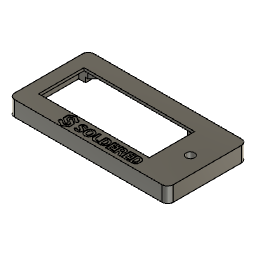
Sensors Case Top (Autodesk Fusion 360 design; units mm, degrees)
Autodesk Fusion 360 part; units mm, degrees
sketch "Sketch1" plane through (0, 0, 0) normal (0, 0, 1) x (1, 0, 0)
  line L0 (65, 35) -> (-65, 35)
  line L1 (-70, 30) -> (-70, -30)
  line L2 (-65, -35) -> (65, -35)
  line L3 (70, -30) -> (70, 30)
  line L4 (70, 35) -> (-70, -35) construction
  line L5 (-70, 35) -> (70, -35) construction
  arc A0 (-65, 35) -> (-70, 30) centre (-65, 30) ccw
  arc A1 (-70, -30) -> (-65, -35) centre (-65, -30) ccw
  arc A2 (65, -35) -> (70, -30) centre (65, -30) ccw
  arc A3 (70, 30) -> (65, 35) centre (65, 30) ccw
  dimension "d1" = 140
  dimension "d2" = 70
  dimension "d3" = 5
  constraint horizontal L0
  constraint perpendicular L0 L1
  constraint parallel L0 L2
  constraint parallel L1 L3
  constraint coincident L4 origin
  constraint coincident L5 origin
  constraint coincident L5.start L0
  constraint coincident L5.start L1
  constraint tangent L0 A0
  constraint tangent L1 A0
  constraint coincident L4.end L1
  constraint coincident L4.end L2
  constraint tangent L1 A1
  constraint tangent L2 A1
  constraint equal A0 A1
  constraint coincident L5.end L3
  constraint coincident L5.end L2
  constraint tangent L3 A2
  constraint tangent L2 A2
  constraint equal A0 A2
  constraint coincident L4.start L3
  constraint coincident L4.start L0
  constraint tangent L3 A3
  constraint tangent L0 A3
  constraint equal A0 A3
  measures "d1" distance of L4.end L5.end
  measures "d2" distance of L5.start L4.end
  measures "d3" radius of A0
extrude "Extrude1" add sketch "Sketch1" along normal blind 14
sketch "Sketch2" plane through (0, 0, 0) normal (0, 0, -1) x (1, 0, 0)
  arc A0 (65, -35) -> (70, -30) centre (65, -30) ccw
  line L0 (70, -30) -> (70, 30)
  arc A1 (70, 30) -> (65, 35) centre (65, 30) ccw
  line L1 (65, 35) -> (-65, 35)
  line L2 (-65, -35) -> (65, -35)
  line L3 (-70, -30) -> (-70, 30)
  line L4 (38.8, 20) -> (-58.8, 20)
  line L5 (-58.8, 20) -> (-58.8, -20)
  line L6 (-58.8, -20) -> (38.8, -20)
  line L7 (38.8, -20) -> (38.8, 20)
  line L8 (38.8, 20) -> (-58.8, -20) construction
  line L9 (-58.8, 20) -> (38.8, -20) construction
  circle A2 centre (-56.6, -27.5) radius 1.6
  circle A3 centre (-56.6, 27.5) radius 2
  circle A4 centre (36.6, 27.5) radius 2
  circle A5 centre (36.6, -27.5) radius 2
  line L10 (39.1, 30) -> (-59.1, 30)
  line L11 (-59.1, 30) -> (-59.1, -30)
  line L12 (-59.1, -30) -> (39.1, -30)
  line L13 (39.1, -30) -> (39.1, 30)
  line L14 (39.1, 30) -> (-59.1, -30) construction
  line L15 (-59.1, 30) -> (39.1, -30) construction
  point P0 (-10, 0)
  point P1 (-10, 0)
  dimension "d70" = 97.6
  dimension "d71" = 40
  dimension "d72" = 3.2
  dimension "d76" = 4
  dimension "d79" = 4
  dimension "d82" = 4
  dimension "d115" = 60
  dimension "d116" = 98.2
  dimension "d117" = 60
  dimension "d118" = 2.5
  dimension "d119" = 2.5
  dimension "d120" = 2.5
  dimension "d121" = 2.5
  dimension "d122" = 2.5
  dimension "d123" = 2.5
  dimension "d124" = 2.5
  dimension "d125" = 2.5
  constraint horizontal L4
  constraint perpendicular L4 L5
  constraint parallel L4 L6
  constraint parallel L5 L7
  constraint coincident L8 P1
  constraint coincident L9 P1
  constraint horizontal L10
  constraint perpendicular L10 L11
  constraint parallel L10 L12
  constraint parallel L11 L13
  constraint coincident L14 P1
  constraint coincident L15 P1
  constraint coincident P1 P0
  measures "d70" distance of L5.end L6.end
  measures "d71" distance of L4.end L5.end
  measures "d72" diameter of A2
  measures "d76" diameter of A3
  measures "d79" diameter of A4
  measures "d82" diameter of A5
  measures "d115" distance of L3 P1
  measures "d116" distance of L11.end L12.end
  measures "d117" distance of L10.end L11.end
  measures "d118" distance of A4.centre L10
  measures "d119" distance of A4.centre L13
  measures "d120" distance of A3.centre L10
  measures "d121" distance of A3.centre L11
  measures "d122" distance of A2.centre L11
  measures "d123" distance of A2.centre L12
  measures "d124" distance of A5.centre L13
  measures "d125" distance of A5.centre L12
extrude "Extrude2" cut sketch "Sketch2" against normal blind 14 contours L4 L5 L6 L7
extrude "Extrude3" cut sketch "Sketch2" against normal blind 8 contours A3 | A4 | A5
sketch "Sketch3" plane through (0, 0, 0) normal (0, 0, -1) x (1, 0, 0)
  arc A0 (65, -35) -> (70, -30) centre (65, -30) ccw
  line L0 (70, -30) -> (70, 30)
  arc A1 (70, 30) -> (65, 35) centre (65, 30) ccw
  line L1 (65, 35) -> (-65, 35)
  arc A2 (-65, 35) -> (-70, 30) centre (-65, 30) ccw
  line L2 (-70, 30) -> (-70, -30)
  arc A3 (-70, -30) -> (-65, -35) centre (-65, -30) ccw
  line L3 (-65, -35) -> (65, -35)
  line L4 (-66, 40) -> (-66, -43.0482) construction
  line L5 (-75, 31) -> (85, 31) construction
  line L6 (66, 43.2494) -> (66, -50) construction
  line L7 (77.8761, -31) -> (-86.4807, -31) construction
  circle A4 centre (-66, -31) radius 2
  circle A5 centre (-66, 31) radius 2
  circle A6 centre (66, 31) radius 2
  circle A7 centre (66, -31) radius 2
  line L8 (38.8, 20) -> (38.8, -20)
  line L9 (38.8, -20) -> (-58.8, -20)
  circle A8 centre (36.6, -27.5) radius 2
  circle A9 centre (36.6, 27.5) radius 2
  circle A10 centre (-56.6, 27.5) radius 2
  line L10 (-58.8, 20) -> (38.8, 20)
  line L11 (-58.8, -20) -> (-58.8, 20)
  dimension "d24" = 4
  dimension "d25" = 4
  dimension "d26" = 4
  dimension "d27" = 4
  dimension "d28" = 4
  dimension "d29" = 4
  dimension "d30" = 4
  dimension "d31" = 4
  constraint perpendicular L1 L4
  constraint perpendicular L4 L5
  constraint perpendicular L3 L6
  constraint perpendicular L6 L7
  constraint coincident L7 A4.centre
  constraint coincident L4 A4.centre
  constraint coincident L4 A5.centre
  constraint coincident L5 A5.centre
  constraint coincident L5 A6.centre
  constraint coincident L6 A6.centre
  constraint coincident L6 A7.centre
  constraint coincident L7 A7.centre
  measures "d24" distance of L2 L4
  measures "d25" distance of L1 L5
  measures "d26" distance of L0 L6
  measures "d27" distance of L3 L7
  measures "d28" diameter of A4
  measures "d29" diameter of A5
  measures "d30" diameter of A6
  measures "d31" diameter of A7
extrude "Extrude4" cut sketch "Sketch3" against normal blind 4 contours A4 | A5 | A6 | A7
sketch "Sketch4" plane through (0, 0, 14) normal (0, 0, 1) x (-1, 0, 0)
  arc A0 (-70, -30) -> (-65, -35) centre (-65, -30) ccw
  line L0 (-65, -35) -> (65, -35)
  arc A1 (65, -35) -> (70, -30) centre (65, -30) ccw
  line L1 (70, -30) -> (70, 30)
  arc A2 (70, 30) -> (65, 35) centre (65, 30) ccw
  line L2 (65, 35) -> (-65, 35)
  arc A3 (-65, 35) -> (-70, 30) centre (-65, 30) ccw
  line L3 (-70, 30) -> (-70, -30)
  circle A4 centre (-55, 0) radius 3.75
  line L4 (-38.8, 20) -> (58.8, 20)
  line L5 (58.8, 20) -> (58.8, -20)
  line L6 (58.8, -20) -> (-38.8, -20)
  line L7 (-38.8, -20) -> (-38.8, 20)
  dimension "d34" = 7.5
  measures "d34" diameter of A4
extrude "Extrude5" cut sketch "Sketch4" against normal blind 10 contours A4
sketch "Sketch5" plane through (0, 0, 0) normal (0, 0, -1) x (1, 0, 0)
  circle A0 centre (66, -31) radius 2
  circle A1 centre (-66, -31) radius 2
  circle A2 centre (66, 31) radius 2
  circle A3 centre (-66, 31) radius 2
  arc A4 (65, -35) -> (70, -30) centre (65, -30) ccw
  line L0 (70, -30) -> (70, 30)
  arc A5 (70, 30) -> (65, 35) centre (65, 30) ccw
  line L1 (65, 35) -> (-65, 35)
  arc A6 (-65, 35) -> (-70, 30) centre (-65, 30) ccw
  line L2 (-70, 30) -> (-70, -30)
  arc A7 (-70, -30) -> (-65, -35) centre (-65, -30) ccw
  line L3 (-65, -35) -> (65, -35)
  line L4 (63, 8) -> (47, 8)
  line L5 (47, 8) -> (47, -8)
  line L6 (47, -8) -> (63, -8)
  line L7 (63, -8) -> (63, 8)
  line L8 (63, 8) -> (47, -8) construction
  line L9 (47, 8) -> (63, -8) construction
  line L10 (38.8, 20) -> (38.8, -20)
  line L11 (38.8, -20) -> (-58.8, -20)
  circle A8 centre (36.6, -27.5) radius 2
  circle A9 centre (36.6, 27.5) radius 2
  circle A10 centre (-56.6, 27.5) radius 2
  line L12 (-58.8, 20) -> (38.8, 20)
  line L13 (-58.8, -20) -> (-58.8, 20)
  point P0 (55, 0)
  dimension "d37" = 16
  dimension "d38" = 16
  constraint horizontal L4
  constraint perpendicular L4 L5
  constraint parallel L4 L6
  constraint parallel L5 L7
  constraint coincident L8 P0
  constraint coincident L9 P0
  measures "d37" distance of L5.end L6.end
  measures "d38" distance of L4.end L5.end
extrude "Extrude6" cut sketch "Sketch5" against normal blind 7 contours L4 L5 L6 L7
chamfer "Chamfer1" distance 2 angle 45 4 edges at (55, -8, 0) (63, 0, 0) (47, 0, 0) (55, 8, 0)
extrude "Extrude7" cut 1 faces at (54.6934, -17.9132, 14) along direction (0, 0, -1) blind 0.6
sketch "Sketch6" plane through (0, 0, 13.4) normal (0, 0, 1) x (-1, 0, 0)
  circle A0 centre (-55, 0) radius 3.75
  arc A1 (-70, -30) -> (-65, -35) centre (-65, -30) ccw
  line L0 (-65, -35) -> (65, -35)
  arc A2 (65, -35) -> (70, -30) centre (65, -30) ccw
  line L1 (70, -30) -> (70, 30)
  arc A3 (70, 30) -> (65, 35) centre (65, 30) ccw
  line L2 (65, 35) -> (-65, 35)
  arc A4 (-65, 35) -> (-70, 30) centre (-65, 30) ccw
  line L3 (-70, 30) -> (-70, -30)
  spline S0 degree 3 poles (14.0223, 31.6995) (14.566, 31.6995) (15.1035, 31.6031) (15.6345, 31.4109) knots 0 0 0 0 1 1 1 1
  spline S1 degree 3 poles (15.6345, 31.4109) (16.1658, 31.2184) (16.649, 30.9174) (17.0838, 30.5076) knots 0 0 0 0 1 1 1 1
  line L4 (17.0838, 30.5076) -> (16.0297, 29.2151)
  spline S2 degree 3 poles (16.0297, 29.2151) (15.737, 29.4578) (15.4068, 29.6438) (15.0385, 29.7734) knots 0 0 0 0 1 1 1 1
  spline S3 degree 3 poles (15.0385, 29.7734) (14.6706, 29.9032) (14.3152, 29.9679) (13.9721, 29.9679) knots 0 0 0 0 1 1 1 1
  spline S4 degree 3 poles (13.9721, 29.9679) (13.6207, 29.9679) (13.3594, 29.9095) (13.1877, 29.7924) knots 0 0 0 0 1 1 1 1
  spline S5 degree 3 poles (13.1877, 29.7924) (13.0165, 29.6752) (12.9306, 29.508) (12.9306, 29.2905) knots 0 0 0 0 1 1 1 1
  spline S6 degree 3 poles (12.9306, 29.2905) (12.9306, 29.1315) (12.9787, 29.0062) (13.0749, 28.9139) knots 0 0 0 0 1 1 1 1
  spline S7 degree 3 poles (13.0749, 28.9139) (13.1712, 28.822) (13.3028, 28.7384) (13.4703, 28.6631) knots 0 0 0 0 1 1 1 1
  spline S8 degree 3 poles (13.4703, 28.6631) (13.6376, 28.5877) (13.8382, 28.5043) (14.0723, 28.412) knots 0 0 0 0 1 1 1 1
  line L5 (14.0723, 28.412) -> (15.1139, 27.973)
  spline S9 degree 3 poles (15.1139, 27.973) (15.4068, 27.8557) (15.6784, 27.6968) (15.9295, 27.4962) knots 0 0 0 0 1 1 1 1
  spline S10 degree 3 poles (15.9295, 27.4962) (16.1803, 27.2954) (16.3833, 27.0465) (16.538, 26.7496) knots 0 0 0 0 1 1 1 1
  spline S11 degree 3 poles (16.538, 26.7496) (16.6928, 26.4528) (16.77, 26.1076) (16.77, 25.7143) knots 0 0 0 0 1 1 1 1
  spline S12 degree 3 poles (16.77, 25.7143) (16.77, 25.2544) (16.6426, 24.8383) (16.3873, 24.4661) knots 0 0 0 0 1 1 1 1
  spline S13 degree 3 poles (16.3873, 24.4661) (16.1324, 24.0937) (15.7811, 23.7947) (15.3335, 23.5687) knots 0 0 0 0 1 1 1 1
  spline S14 degree 3 poles (15.3335, 23.5687) (14.8861, 23.3431) (14.3695, 23.2299) (13.7839, 23.2299) knots 0 0 0 0 1 1 1 1
  spline S15 degree 3 poles (13.7839, 23.2299) (13.2904, 23.2299) (12.8113, 23.3179) (12.3473, 23.4935) knots 0 0 0 0 1 1 1 1
  spline S16 degree 3 poles (12.3473, 23.4935) (11.8829, 23.6691) (11.475, 23.9243) (11.1238, 24.2588) knots 0 0 0 0 1 1 1 1
  line L6 (11.1238, 24.2588) -> (12.1651, 25.5639)
  spline S17 degree 3 poles (12.1651, 25.5639) (12.4413, 25.363) (12.7152, 25.2124) (12.987, 25.1122) knots 0 0 0 0 1 1 1 1
  spline S18 degree 3 poles (12.987, 25.1122) (13.259, 25.0118) (13.5247, 24.9616) (13.7839, 24.9616) knots 0 0 0 0 1 1 1 1
  spline S19 degree 3 poles (13.7839, 24.9616) (14.0766, 24.9616) (14.3089, 25.0161) (14.4801, 25.1246) knots 0 0 0 0 1 1 1 1
  spline S20 degree 3 poles (14.4801, 25.1246) (14.6518, 25.2335) (14.7376, 25.3925) (14.7376, 25.6014) knots 0 0 0 0 1 1 1 1
  spline S21 degree 3 poles (14.7376, 25.6014) (14.7376, 25.7437) (14.6873, 25.865) (14.5869, 25.9654) knots 0 0 0 0 1 1 1 1
  spline S22 degree 3 poles (14.5869, 25.9654) (14.4865, 26.0658) (14.3422, 26.1535) (14.154, 26.2289) knots 0 0 0 0 1 1 1 1
  spline S23 degree 3 poles (14.154, 26.2289) (13.9657, 26.3042) (13.7505, 26.3919) (13.5078, 26.4924) knots 0 0 0 0 1 1 1 1
  line L7 (13.5078, 26.4924) -> (12.4916, 26.8938)
  spline S24 degree 3 poles (12.4916, 26.8938) (12.157, 27.0277) (11.8704, 27.1972) (11.632, 27.402) knots 0 0 0 0 1 1 1 1
  spline S25 degree 3 poles (11.632, 27.402) (11.3936, 27.607) (11.2098, 27.8497) (11.0799, 28.1297) knots 0 0 0 0 1 1 1 1
  spline S26 degree 3 poles (11.0799, 28.1297) (10.9503, 28.4102) (10.8854, 28.7427) (10.8854, 29.1271) knots 0 0 0 0 1 1 1 1
  spline S27 degree 3 poles (10.8854, 29.1271) (10.8854, 29.5875) (11.0066, 30.0118) (11.2493, 30.4008) knots 0 0 0 0 1 1 1 1
  spline S28 degree 3 poles (11.2493, 30.4008) (11.492, 30.7898) (11.8474, 31.1036) (12.3157, 31.342) knots 0 0 0 0 1 1 1 1
  spline S29 degree 3 poles (12.3157, 31.342) (12.7845, 31.5804) (13.3531, 31.6995) (14.0223, 31.6995) knots 0 0 0 0 1 1 1 1
  spline S30 degree 3 poles (6.5316, 29.9679) (6.1801, 29.9679) (5.8771, 29.8657) (5.6219, 29.6605) knots 0 0 0 0 1 1 1 1
  spline S31 degree 3 poles (5.6219, 29.6605) (5.3668, 29.4556) (5.1723, 29.163) (5.0384, 28.7822) knots 0 0 0 0 1 1 1 1
  spline S32 degree 3 poles (5.0384, 28.7822) (4.9046, 28.4016) (4.8377, 27.9521) (4.8377, 27.4333) knots 0 0 0 0 1 1 1 1
  spline S33 degree 3 poles (4.8377, 27.4333) (4.8377, 26.9063) (4.9046, 26.4609) (5.0384, 26.097) knots 0 0 0 0 1 1 1 1
  spline S34 degree 3 poles (5.0384, 26.097) (5.1723, 25.7333) (5.3668, 25.4531) (5.6219, 25.2563) knots 0 0 0 0 1 1 1 1
  spline S35 degree 3 poles (5.6219, 25.2563) (5.8771, 25.06) (6.1801, 24.9616) (6.5316, 24.9616) knots 0 0 0 0 1 1 1 1
  spline S36 degree 3 poles (6.5316, 24.9616) (6.8829, 24.9616) (7.1862, 25.06) (7.4413, 25.2563) knots 0 0 0 0 1 1 1 1
  spline S37 degree 3 poles (7.4413, 25.2563) (7.6964, 25.4531) (7.8909, 25.7333) (8.0247, 26.097) knots 0 0 0 0 1 1 1 1
  spline S38 degree 3 poles (8.0247, 26.097) (8.1586, 26.4609) (8.2255, 26.9063) (8.2255, 27.4333) knots 0 0 0 0 1 1 1 1
  spline S39 degree 3 poles (8.2255, 27.4333) (8.2255, 27.9521) (8.1586, 28.4016) (8.0247, 28.7822) knots 0 0 0 0 1 1 1 1
  spline S40 degree 3 poles (8.0247, 28.7822) (7.8909, 29.163) (7.6964, 29.4556) (7.4413, 29.6605) knots 0 0 0 0 1 1 1 1
  spline S41 degree 3 poles (7.4413, 29.6605) (7.1862, 29.8657) (6.8829, 29.9679) (6.5316, 29.9679) knots 0 0 0 0 1 1 1 1
  spline S42 degree 3 poles (6.5316, 31.6996) (7.2762, 31.6996) (7.9305, 31.5301) (8.4953, 31.1913) knots 0 0 0 0 1 1 1 1
  spline S43 degree 3 poles (8.4953, 31.1913) (9.0598, 30.8525) (9.4989, 30.3632) (9.8126, 29.7232) knots 0 0 0 0 1 1 1 1
  spline S44 degree 3 poles (9.8126, 29.7232) (10.1263, 29.0833) (10.2833, 28.3201) (10.2833, 27.4333) knots 0 0 0 0 1 1 1 1
  spline S45 degree 3 poles (10.2833, 27.4333) (10.2833, 26.5383) (10.1263, 25.7792) (9.8126, 25.1561) knots 0 0 0 0 1 1 1 1
  spline S46 degree 3 poles (9.8126, 25.1561) (9.4989, 24.533) (9.0598, 24.0561) (8.4953, 23.7257) knots 0 0 0 0 1 1 1 1
  spline S47 degree 3 poles (8.4953, 23.7257) (7.9305, 23.3953) (7.2762, 23.2299) (6.5316, 23.2299) knots 0 0 0 0 1 1 1 1
  spline S48 degree 3 poles (6.5316, 23.2299) (5.7872, 23.2299) (5.1325, 23.3953) (4.5678, 23.7257) knots 0 0 0 0 1 1 1 1
  spline S49 degree 3 poles (4.5678, 23.7257) (4.0034, 24.0561) (3.5641, 24.533) (3.2503, 25.1561) knots 0 0 0 0 1 1 1 1
  spline S50 degree 3 poles (3.2503, 25.1561) (2.9367, 25.7792) (2.7799, 26.5383) (2.7799, 27.4333) knots 0 0 0 0 1 1 1 1
  spline S51 degree 3 poles (2.7799, 27.4333) (2.7799, 28.3201) (2.9367, 29.0833) (3.2503, 29.7232) knots 0 0 0 0 1 1 1 1
  spline S52 degree 3 poles (3.2503, 29.7232) (3.5641, 30.3632) (4.0034, 30.8525) (4.5678, 31.1913) knots 0 0 0 0 1 1 1 1
  spline S53 degree 3 poles (4.5678, 31.1913) (5.1325, 31.5301) (5.7872, 31.6996) (6.5316, 31.6996) knots 0 0 0 0 1 1 1 1
  line L8 (-6.2916, 29.9428) -> (-6.53, 29.9428)
  spline S54 degree 3 poles (-6.53, 29.9428) (-6.9565, 29.9428) (-7.3373, 29.8675) (-7.6717, 29.7171) knots 0 0 0 0 1 1 1 1
  spline S55 degree 3 poles (-7.6717, 29.7171) (-8.0063, 29.5665) (-8.2698, 29.3093) (-8.4623, 28.9452) knots 0 0 0 0 1 1 1 1
  spline S56 degree 3 poles (-8.4623, 28.9452) (-8.6546, 28.5814) (-8.7508, 28.0777) (-8.7508, 27.4332) knots 0 0 0 0 1 1 1 1
  spline S57 degree 3 poles (-8.7508, 27.4332) (-8.7508, 26.7894) (-8.6546, 26.2916) (-8.4623, 25.9403) knots 0 0 0 0 1 1 1 1
  spline S58 degree 3 poles (-8.4623, 25.9403) (-8.2698, 25.589) (-8.0063, 25.3422) (-7.6717, 25.2) knots 0 0 0 0 1 1 1 1
  spline S59 degree 3 poles (-7.6717, 25.2) (-7.3373, 25.0577) (-6.9565, 24.9867) (-6.53, 24.9867) knots 0 0 0 0 1 1 1 1
  line L9 (-6.53, 24.9867) -> (-6.2916, 24.9867)
  line L10 (-6.2916, 24.9867) -> (-6.2916, 29.9428)
  line L11 (-4.284, 31.5489) -> (-4.284, 23.3806)
  line L12 (-4.284, 23.3806) -> (-6.6555, 23.3806)
  spline S60 degree 3 poles (-6.6555, 23.3806) (-7.4836, 23.3806) (-8.2092, 23.5208) (-8.8325, 23.8008) knots 0 0 0 0 1 1 1 1
  spline S61 degree 3 poles (-8.8325, 23.8008) (-9.4555, 24.0812) (-9.9386, 24.5182) (-10.2818, 25.1122) knots 0 0 0 0 1 1 1 1
  spline S62 degree 3 poles (-10.2818, 25.1122) (-10.6246, 25.7062) (-10.796, 26.4797) (-10.796, 27.4332) knots 0 0 0 0 1 1 1 1
  spline S63 degree 3 poles (-10.796, 27.4332) (-10.796, 28.3787) (-10.6246, 29.1546) (-10.2818, 29.761) knots 0 0 0 0 1 1 1 1
  spline S64 degree 3 poles (-10.2818, 29.761) (-9.9386, 30.3675) (-9.4641, 30.817) (-8.8576, 31.1097) knots 0 0 0 0 1 1 1 1
  spline S65 degree 3 poles (-8.8576, 31.1097) (-8.251, 31.4026) (-7.5547, 31.5489) (-6.7684, 31.5489) knots 0 0 0 0 1 1 1 1
  line L13 (-6.7684, 31.5489) -> (-4.284, 31.5489)
  line L14 (-11.7133, 31.5489) -> (-11.7133, 23.3806)
  line L15 (-11.7133, 23.3806) -> (-16.9204, 23.3806)
  line L16 (-16.9204, 23.3806) -> (-16.9204, 25.0619)
  line L17 (-16.9204, 25.0619) -> (-13.7209, 25.0619)
  line L18 (-13.7209, 25.0619) -> (-13.7209, 26.5174)
  line L19 (-13.7209, 26.5174) -> (-16.4437, 26.5174)
  line L20 (-16.4437, 26.5174) -> (-16.4437, 28.1987)
  line L21 (-16.4437, 28.1987) -> (-13.7209, 28.1987)
  line L22 (-13.7209, 28.1987) -> (-13.7209, 29.8675)
  line L23 (-13.7209, 29.8675) -> (-17.0459, 29.8675)
  line L24 (-17.0459, 29.8675) -> (-17.0459, 31.5489)
  line L25 (-17.0459, 31.5489) -> (-11.7133, 31.5489)
  line L26 (-20.145, 24.974) -> (-21.0109, 24.974)
  spline S66 degree 3 poles (-21.0109, 24.974) (-21.4625, 24.974) (-21.8074, 25.0452) (-22.0458, 25.1873) knots 0 0 0 0 1 1 1 1
  spline S67 degree 3 poles (-22.0458, 25.1873) (-22.2843, 25.3297) (-22.4035, 25.5933) (-22.4035, 25.9778) knots 0 0 0 0 1 1 1 1
  spline S68 degree 3 poles (-22.4035, 25.9778) (-22.4035, 26.3544) (-22.2843, 26.6388) (-22.0458, 26.8312) knots 0 0 0 0 1 1 1 1
  spline S69 degree 3 poles (-22.0458, 26.8312) (-21.8074, 27.0237) (-21.4625, 27.1196) (-21.0109, 27.1196) knots 0 0 0 0 1 1 1 1
  line L27 (-21.0109, 27.1196) -> (-20.145, 27.1196)
  line L28 (-20.145, 27.1196) -> (-20.145, 24.974)
  line L29 (-24.7876, 31.5489) -> (-22.974, 28.3209)
  spline S70 degree 3 poles (-22.974, 28.3209) (-23.3572, 28.1311) (-23.678, 27.8717) (-23.9282, 27.5337) knots 0 0 0 0 1 1 1 1
  spline S71 degree 3 poles (-23.9282, 27.5337) (-24.225, 27.1323) (-24.3736, 26.6136) (-24.3736, 25.9778) knots 0 0 0 0 1 1 1 1
  spline S72 degree 3 poles (-24.3736, 25.9778) (-24.3736, 25.3088) (-24.225, 24.7858) (-23.9282, 24.4094) knots 0 0 0 0 1 1 1 1
  spline S73 degree 3 poles (-23.9282, 24.4094) (-23.631, 24.0331) (-23.2399, 23.7676) (-22.7549, 23.6127) knots 0 0 0 0 1 1 1 1
  spline S74 degree 3 poles (-22.7549, 23.6127) (-22.2696, 23.4579) (-21.7385, 23.3806) (-21.1615, 23.3806) knots 0 0 0 0 1 1 1 1
  line L30 (-21.1615, 23.3806) -> (-18.1375, 23.3806)
  line L31 (-18.1375, 23.3806) -> (-18.1375, 31.5489)
  line L32 (-18.1375, 31.5489) -> (-20.145, 31.5489)
  line L33 (-20.145, 31.5489) -> (-20.145, 28.7133)
  line L34 (-20.145, 28.7133) -> (-21.0729, 28.7133)
  line L35 (-21.0729, 28.7133) -> (-22.5541, 31.5489)
  line L36 (-22.5541, 31.5489) -> (-24.7876, 31.5489)
  line L37 (-25.5653, 31.5489) -> (-25.5653, 23.3806)
  line L38 (-25.5653, 23.3806) -> (-30.7725, 23.3806)
  line L39 (-30.7725, 23.3806) -> (-30.7725, 25.0619)
  line L40 (-30.7725, 25.0619) -> (-27.5728, 25.0619)
  line L41 (-27.5728, 25.0619) -> (-27.5728, 26.5174)
  line L42 (-27.5728, 26.5174) -> (-30.2957, 26.5174)
  line L43 (-30.2957, 26.5174) -> (-30.2957, 28.1987)
  line L44 (-30.2957, 28.1987) -> (-27.5728, 28.1987)
  line L45 (-27.5728, 28.1987) -> (-27.5728, 29.8675)
  line L46 (-27.5728, 29.8675) -> (-30.8979, 29.8675)
  line L47 (-30.8979, 29.8675) -> (-30.8979, 31.5489)
  line L48 (-30.8979, 31.5489) -> (-25.5653, 31.5489)
  line L49 (-33.8716, 29.9428) -> (-34.11, 29.9428)
  spline S75 degree 3 poles (-34.11, 29.9428) (-34.5366, 29.9428) (-34.9173, 29.8675) (-35.2518, 29.7171) knots 0 0 0 0 1 1 1 1
  spline S76 degree 3 poles (-35.2518, 29.7171) (-35.5863, 29.5665) (-35.8499, 29.3093) (-36.0423, 28.9452) knots 0 0 0 0 1 1 1 1
  spline S77 degree 3 poles (-36.0423, 28.9452) (-36.2346, 28.5814) (-36.3309, 28.0777) (-36.3309, 27.4332) knots 0 0 0 0 1 1 1 1
  spline S78 degree 3 poles (-36.3309, 27.4332) (-36.3309, 26.7894) (-36.2346, 26.2916) (-36.0423, 25.9403) knots 0 0 0 0 1 1 1 1
  spline S79 degree 3 poles (-36.0423, 25.9403) (-35.8499, 25.589) (-35.5863, 25.3422) (-35.2518, 25.2) knots 0 0 0 0 1 1 1 1
  spline S80 degree 3 poles (-35.2518, 25.2) (-34.9173, 25.0577) (-34.5366, 24.9867) (-34.11, 24.9867) knots 0 0 0 0 1 1 1 1
  line L50 (-34.11, 24.9867) -> (-33.8716, 24.9867)
  line L51 (-33.8716, 24.9867) -> (-33.8716, 29.9428)
  line L52 (-31.8641, 31.5489) -> (-31.8641, 23.3806)
  line L53 (-31.8641, 23.3806) -> (-34.2355, 23.3806)
  spline S81 degree 3 poles (-34.2355, 23.3806) (-35.0636, 23.3806) (-35.7892, 23.5208) (-36.4126, 23.8008) knots 0 0 0 0 1 1 1 1
  spline S82 degree 3 poles (-36.4126, 23.8008) (-37.0355, 24.0812) (-37.5186, 24.5182) (-37.8618, 25.1122) knots 0 0 0 0 1 1 1 1
  spline S83 degree 3 poles (-37.8618, 25.1122) (-38.2046, 25.7062) (-38.376, 26.4797) (-38.376, 27.4332) knots 0 0 0 0 1 1 1 1
  spline S84 degree 3 poles (-38.376, 27.4332) (-38.376, 28.3787) (-38.2046, 29.1546) (-37.8618, 29.761) knots 0 0 0 0 1 1 1 1
  spline S85 degree 3 poles (-37.8618, 29.761) (-37.5186, 30.3675) (-37.0441, 30.817) (-36.4376, 31.1097) knots 0 0 0 0 1 1 1 1
  spline S86 degree 3 poles (-36.4376, 31.1097) (-35.831, 31.4026) (-35.1347, 31.5489) (-34.3485, 31.5489) knots 0 0 0 0 1 1 1 1
  line L54 (-34.3485, 31.5489) -> (-31.8641, 31.5489)
  line L55 (-1.2206, 29.5917) -> (-0.0935, 28.4645)
  line L56 (-0.0935, 28.4645) -> (-0.0935, 23.3806)
  line L57 (-0.0935, 23.3806) -> (1.9141, 23.3806)
  line L58 (1.9141, 23.3806) -> (1.9141, 29.4411)
  line L59 (1.9141, 29.4411) -> (-0.1704, 31.5255)
  line L60 (-0.1704, 31.5255) -> (-3.3165, 31.5255)
  line L61 (-3.3165, 31.5255) -> (-3.3165, 29.5917)
  line L62 (-3.3165, 29.5917) -> (-1.2206, 29.5917)
  line L63 (21.169, 22.4657) -> (21.1725, 22.4657)
  spline S87 degree 3 poles (21.1725, 22.4657) (21.4299, 22.4663) (21.6835, 22.4038) (21.9065, 22.2751) knots 0 0 0 0 1 1 1 1
  line L64 (21.9065, 22.2751) -> (25.0192, 20.478)
  line L65 (25.0192, 20.478) -> (29.6844, 23.1693)
  line L66 (29.6844, 23.1693) -> (29.6844, 27.7005)
  line L67 (29.6844, 27.7005) -> (24.7789, 30.5327)
  line L68 (24.7789, 30.5327) -> (24.665, 30.4733)
  spline S88 degree 3 poles (24.665, 30.4733) (24.2399, 30.2534) (23.9257, 29.7858) (23.919, 29.3072) knots 0 0 0 0 1 1 1 1
  spline S89 degree 3 poles (23.919, 29.3072) (23.9121, 28.8287) (24.2143, 28.292) (24.6326, 28.0603) knots 0 0 0 0 1 1 1 1
  line L69 (24.6326, 28.0603) -> (27.5947, 26.4695)
  line L70 (27.5947, 26.4695) -> (27.5947, 24.3462)
  line L71 (27.5947, 24.3462) -> (25.0293, 22.8515)
  line L72 (25.0293, 22.8515) -> (22.8789, 24.1087)
  spline S90 degree 3 poles (22.8789, 24.1087) (22.6755, 24.2276) (22.5102, 24.3999) (22.3905, 24.6028) knots 0 0 0 0 1 1 1 1
  spline S91 degree 3 poles (22.3905, 24.6028) (22.1439, 25.0206) (21.6892, 25.301) (21.169, 25.301) knots 0 0 0 0 1 1 1 1
  spline S92 degree 3 poles (21.169, 25.301) (20.6954, 25.301) (20.2764, 25.0686) (20.0189, 24.7118) knots 0 0 0 0 1 1 1 1
  spline S93 degree 3 poles (20.0189, 24.7118) (19.9943, 24.6789) (19.971, 24.6443) (19.95, 24.6077) knots 0 0 0 0 1 1 1 1
  spline S94 degree 3 poles (19.95, 24.6077) (19.9472, 24.603) (19.9448, 24.5983) (19.9423, 24.5935) knots 0 0 0 0 1 1 1 1
  spline S95 degree 3 poles (19.9423, 24.5935) (19.8211, 24.3846) (19.7514, 24.1422) (19.7514, 23.8833) knots 0 0 0 0 1 1 1 1
  spline S96 degree 3 poles (19.7514, 23.8833) (19.7514, 23.1005) (20.386, 22.4657) (21.169, 22.4657) knots 0 0 0 0 1 1 1 1
  spline S97 degree 3 poles (25.2044, 24.2526) (25.6294, 24.4726) (25.9437, 24.9401) (25.9505, 25.4187) knots 0 0 0 0 1 1 1 1
  spline S98 degree 3 poles (25.9505, 25.4187) (25.9573, 25.8972) (25.6551, 26.434) (25.2368, 26.6656) knots 0 0 0 0 1 1 1 1
  line L73 (25.2368, 26.6656) -> (22.2747, 28.2565)
  line L74 (22.2747, 28.2565) -> (22.2747, 30.3797)
  line L75 (22.2747, 30.3797) -> (24.8401, 31.8744)
  line L76 (24.8401, 31.8744) -> (26.9905, 30.6172)
  spline S99 degree 3 poles (26.9905, 30.6172) (27.1939, 30.4984) (27.3593, 30.3262) (27.4789, 30.1232) knots 0 0 0 0 1 1 1 1
  spline S100 degree 3 poles (27.4789, 30.1232) (27.7255, 29.7053) (28.1801, 29.425) (28.7004, 29.425) knots 0 0 0 0 1 1 1 1
  spline S101 degree 3 poles (28.7004, 29.425) (29.174, 29.425) (29.593, 29.6574) (29.8504, 30.0141) knots 0 0 0 0 1 1 1 1
  spline S102 degree 3 poles (29.8504, 30.0141) (29.8751, 30.0471) (29.8983, 30.0816) (29.9194, 30.1182) knots 0 0 0 0 1 1 1 1
  spline S103 degree 3 poles (29.9194, 30.1182) (29.9222, 30.123) (29.9245, 30.1277) (29.9271, 30.1323) knots 0 0 0 0 1 1 1 1
  spline S104 degree 3 poles (29.9271, 30.1323) (30.0483, 30.3413) (30.118, 30.5837) (30.118, 30.8426) knots 0 0 0 0 1 1 1 1
  spline S105 degree 3 poles (30.118, 30.8426) (30.118, 31.6256) (29.4833, 32.2602) (28.7004, 32.2602) knots 0 0 0 0 1 1 1 1
  line L77 (28.7004, 32.2602) -> (28.697, 32.2602)
  spline S106 degree 3 poles (28.697, 32.2602) (28.4394, 32.2596) (28.1858, 32.3221) (27.9629, 32.4508) knots 0 0 0 0 1 1 1 1
  line L78 (27.9629, 32.4508) -> (24.8502, 34.248)
  line L79 (24.8502, 34.248) -> (20.1849, 31.5566)
  line L80 (20.1849, 31.5566) -> (20.1849, 27.0255)
  line L81 (20.1849, 27.0255) -> (25.0905, 24.1932)
  line L82 (25.0905, 24.1932) -> (25.2044, 24.2526)
  line L83 (-38.8, 20) -> (58.8, 20)
  line L84 (58.8, 20) -> (58.8, -20)
  line L85 (58.8, -20) -> (-38.8, -20)
  line L86 (-38.8, -20) -> (-38.8, 20)
extrude "Extrude8" cut sketch "Sketch6" against normal blind 0.5 contours S0 S1 L4 S2 S3 S4 S5 S6 S7 S8 L5 S9 S10 S11 S12 S13 S14 S15 S16 L6 S17 S18 S19 S20 S21 S22 S23 L7 S24 S25 S26 S27 S28 S29 | S42 S43 S44 S45 S46 S47 S48 S49 S50 S51 S52 S53 | L11 L12 S60 S61 S62 S63 S64 S65 L13 | L14 L15 L16 L17 L18 L19 L20 L21 L22 L23 L24 L25 | L29 S70 S71 S72 S73 S74 L30 L31 L32 L33 L34 L35 L36 | L37 L38 L39 L40 L41 L42 L43 L44 L45 L46 L47 L48 | L52 L53 S81 S82 S83 S84 S85 S86 L54 | L55 L56 L57 L58 L59 L60 L61 L62 | L63 S87 L64 L65 L66 L67 L68 S88 S89 L69 L70 L71 L72 S90 S91 S92 S93 S94 S95 S96 | S97 S98 L73 L74 L75 L76 S99 S100 S101 S102 S103 S104 S105 L77 S106 L78 L79 L80 L81 L82
sketch "Sketch7" plane through (0, 0, 0) normal (0, 0, -1) x (1, 0, 0)
  arc A0 (65, -35) -> (70, -30) centre (65, -30) ccw
  line L0 (70, -30) -> (70, 30)
  arc A1 (70, 30) -> (65, 35) centre (65, 30) ccw
  line L1 (65, 35) -> (-65, 35)
  arc A2 (-65, 35) -> (-70, 30) centre (-65, 30) ccw
  line L2 (-70, 30) -> (-70, -30)
  arc A3 (-70, -30) -> (-65, -35) centre (-65, -30) ccw
  line L3 (-65, -35) -> (65, -35)
  circle A4 centre (-66, 31) radius 2
  circle A5 centre (66, 31) radius 2
  circle A6 centre (-66, -31) radius 2
  circle A7 centre (66, -31) radius 2
  line L4 (45, 10) -> (65, 10)
  line L5 (65, 10) -> (65, -10)
  line L6 (65, -10) -> (45, -10)
  line L7 (45, -10) -> (45, 10)
  line L8 (60, 22.5) -> (-60, 22.5)
  line L9 (-60, 22.5) -> (-60, -22.5)
  line L10 (-60, -22.5) -> (60, -22.5)
  line L11 (60, -22.5) -> (60, 22.5)
  line L12 (60, 22.5) -> (-60, -22.5) construction
  line L13 (-60, 22.5) -> (60, -22.5) construction
  line L14 (-60, 22.5) -> (-66, 22.5)
  line L15 (-66, 22.5) -> (-66, -22.5)
  line L16 (-66, -22.5) -> (-60, -22.5)
  line L17 (-60, -22.5) -> (-60, 22.5)
  line L18 (60, 22.5) -> (66, 22.5)
  line L19 (66, 22.5) -> (66, -22.5)
  line L20 (66, -22.5) -> (60, -22.5)
  line L21 (60, -22.5) -> (60, 22.5)
  line L22 (-25, 30) -> (25, 30)
  line L23 (25, 30) -> (25, 15)
  line L24 (25, 15) -> (-25, 15)
  line L25 (-25, 15) -> (-25, 30)
  line L26 (-25, 30) -> (25, 15) construction
  line L27 (25, 30) -> (-25, 15) construction
  line L28 (-25, 30) -> (-53, 30)
  line L29 (-53, 30) -> (-53, 22.5)
  line L30 (-53, 22.5) -> (-25, 22.5)
  line L31 (-25, 22.5) -> (-25, 30)
  line L32 (0, 0) -> (-17.5095, 0) construction
  line L33 (-53, -30) -> (-53, -22.5)
  line L34 (25, -30) -> (-25, -15) construction
  line L35 (-25, -30) -> (25, -30)
  line L36 (-25, -30) -> (-53, -30)
  line L37 (-25, -22.5) -> (-25, -30)
  line L38 (-25, -15) -> (-25, -30)
  line L39 (25, -30) -> (25, -15)
  line L40 (-53, -22.5) -> (-25, -22.5)
  line L41 (-25, -30) -> (25, -15) construction
  line L42 (25, -15) -> (-25, -15)
  line L43 (38.8, 20) -> (38.8, -20)
  line L44 (38.8, -20) -> (-58.8, -20)
  line L45 (25, 30) -> (60, 30)
  line L46 (60, 30) -> (60, 22.5)
  line L47 (60, 22.5) -> (25, 22.5)
  line L48 (25, 22.5) -> (25, 30)
  line L49 (25, -30) -> (60, -30)
  line L50 (60, -30) -> (60, -22.5)
  line L51 (60, -22.5) -> (25, -22.5)
  line L52 (25, -22.5) -> (25, -30)
  line L53 (-58.8, 20) -> (38.8, 20)
  line L54 (-58.8, -20) -> (-58.8, 20)
  circle A8 centre (-56.6, 27.5) radius 2
  circle A9 centre (36.6, 27.5) radius 2
  circle A10 centre (36.6, -27.5) radius 2
  point P0 (0, 22.5)
  point P1 (0, -22.5)
  dimension "d58" = 6
  dimension "d59" = 45
  dimension "d60" = 6
  dimension "d63" = 45
  dimension "d64" = 120
  dimension "d65" = 45
  dimension "d66" = 28
  constraint horizontal L8
  constraint perpendicular L8 L9
  constraint parallel L8 L10
  constraint parallel L9 L11
  constraint coincident L12 L32.start
  constraint coincident L13 L32.start
  constraint coincident L32.start origin
  constraint horizontal L14
  constraint vertical L15
  constraint horizontal L16
  constraint vertical L17
  constraint horizontal L18
  constraint vertical L19
  constraint horizontal L20
  constraint vertical L21
  constraint horizontal L22
  constraint perpendicular L22 L23
  constraint parallel L22 L24
  constraint parallel L23 L25
  constraint coincident L26 P0
  constraint coincident L27 P0
  constraint midpoint L8 P0
  constraint horizontal L28
  constraint vertical L29
  constraint horizontal L30
  constraint vertical L31
  constraint horizontal L32
  constraint symmetric L22.start L32 L35.start
  constraint symmetric L22.end L32 L34.start
  constraint symmetric L23.end L32 L39.end
  constraint symmetric L24.end L32 L34.end
  constraint symmetric P0 L32 P1
  constraint symmetric L28.end L32 L33.start
  constraint symmetric L29.end L32 L33.end
  constraint symmetric L30.end L32 L37.start
  constraint horizontal L45
  constraint vertical L46
  constraint horizontal L47
  constraint vertical L48
  constraint horizontal L49
  constraint vertical L50
  constraint horizontal L51
  constraint vertical L52
  measures "d58" distance of L8.end L14.end
  measures "d59" distance of L8.end L9.end
  measures "d60" distance of L8.start L18.end
  measures "d63" distance of L8.end L9.end
  measures "d64" distance of L9.end L10.end
  measures "d65" distance of L18.end L19.end
  measures "d66" distance of L22.start L28.end
extrude "Extrude9" cut sketch "Sketch7" against normal blind 8 contours L4 L6 L7 L8 L10 L11 L21 L23 L39 L43 L44 L47 L51 L53 | L4 L6 L7 L11 L21 | L4 L5 L6 L11 L18 L19 L20 L21 | L4 L5 L6 L11 L21 | L8 L23 L25 L53 | L8 L22 L23 L25 L31 L48 | L10 L35 L37 L38 L39 L52 | L10 L38 L39 L44 | L8 L9 L10 L17 L25 L30 L38 L40 L44 L53 L54 | L8 L25 L28 L29 L30 L31 | L23 L24 L25 L38 L39 L42 L43 L44 L53 L54 | L23 L24 L25 L53 | L10 L33 L36 L37 L38 L40 | L38 L39 L42 L44 | L9 L14 L15 L16 L17
chamfer "Chamfer2" distance 5 angle 45 4 edges at (-53, -22.5, 4) (25, -22.5, 4) (-53, 22.5, 4) (25, 22.5, 4)
sketch "Sketch14" plane through (0, 0, 8) normal (0, 0, -1) x (1, 0, 0)
  line L0 (-66, -22.5) -> (-58, -22.5)
  line L1 (66, -22.5) -> (66, 22.5)
  line L2 (-58, 22.5) -> (-66, 22.5)
  line L3 (62, 7) -> (60, 7)
  line L4 (60, 7) -> (60, 5)
  line L5 (60, 5) -> (62, 5)
  line L6 (62, 5) -> (62, 7)
  line L7 (62, 7) -> (60, 5) construction
  line L8 (60, 7) -> (62, 5) construction
  line L9 (60, 6.3) -> (61.3, 6.3)
  line L10 (61.3, 5) -> (61.3, 6.3)
  line L11 (55, 0) -> (62, 0) construction
  line L12 (55, 0) -> (55, 7) construction
  line L13 (50, 6.3) -> (48.7, 6.3)
  line L14 (50, 5) -> (48, 5)
  line L15 (48, 7) -> (50, 5) construction
  line L16 (48.7, 5) -> (48.7, 6.3)
  line L17 (50, 7) -> (48, 5) construction
  line L18 (48, 7) -> (50, 7)
  line L19 (50, 7) -> (50, 5)
  line L20 (48, 5) -> (48, 7)
  line L21 (48.7, -5) -> (48.7, -6.3)
  line L22 (50, -6.3) -> (48.7, -6.3)
  line L23 (50, -5) -> (48, -5)
  line L24 (50, -7) -> (48, -5) construction
  line L25 (48, -7) -> (50, -7)
  line L26 (50, -7) -> (50, -5)
  line L27 (48, -5) -> (48, -7)
  line L28 (48, -7) -> (50, -5) construction
  line L29 (62, -7) -> (60, -7)
  line L30 (61.3, -5) -> (61.3, -6.3)
  line L31 (60, -7) -> (62, -5) construction
  line L32 (62, -5) -> (62, -7)
  line L33 (60, -7) -> (60, -5)
  line L34 (62, -7) -> (60, -5) construction
  line L35 (60, -5) -> (62, -5)
  line L36 (60, -6.3) -> (61.3, -6.3)
  line L37 (38.8, 20) -> (38.8, -20)
  line L38 (38.8, -20) -> (-58.8, -20)
  circle A0 centre (55, 0) radius 3.75
  line L39 (-58.8, -20) -> (-58.8, 20)
  line L40 (-58.8, 20) -> (38.8, 20)
  line L41 (-66, 22.5) -> (-66, -22.5)
  line L42 (-58, -22.5) -> (-53, -27.5)
  line L43 (-53, -27.5) -> (-53, -30)
  line L44 (-53, -30) -> (25, -30)
  line L45 (25, -30) -> (25, -27.5)
  line L46 (25, -27.5) -> (30, -22.5)
  line L47 (25, 27.5) -> (25, 30)
  line L48 (25, 30) -> (-53, 30)
  line L49 (-53, 30) -> (-53, 27.5)
  line L50 (-53, 27.5) -> (-58, 22.5)
  line L51 (30, 22.5) -> (25, 27.5)
  line L52 (30, -22.5) -> (66, -22.5)
  line L53 (66, 22.5) -> (30, 22.5)
  line L54 (62, 5) -> (61.3, 5)
  line L55 (61.3, 5) -> (61.3, -5)
  line L56 (61.3, -5) -> (62, -5)
  line L57 (62, -5) -> (62, 5)
  line L58 (60, -6.3) -> (50, -6.3)
  line L59 (50, -6.3) -> (50, -7)
  line L60 (50, -7) -> (60, -7)
  line L61 (60, -7) -> (60, -6.3)
  line L62 (48.7, -5) -> (48, -5)
  line L63 (48, -5) -> (48, 5)
  line L64 (48, 5) -> (48.7, 5)
  line L65 (48.7, 5) -> (48.7, -5)
  line L66 (50, 6.3) -> (60, 6.3)
  line L67 (60, 6.3) -> (60, 7)
  line L68 (60, 7) -> (50, 7)
  line L69 (50, 7) -> (50, 6.3)
  point P0 (61, 6)
  point P1 (49, 6)
  point P2 (49, -6)
  point P3 (61, -6)
  dimension "d100" = 0.7
  constraint horizontal L3
  constraint perpendicular L3 L4
  constraint parallel L3 L5
  constraint parallel L4 L6
  constraint coincident L7 P0
  constraint coincident L8 P0
  constraint coincident L4 L9.start
  constraint coincident L7 L9.end
  constraint perpendicular L4 L9
  constraint coincident L5 L10.start
  constraint perpendicular L9 L10
  constraint horizontal L11
  constraint perpendicular L11 L12
  constraint symmetric L3.start L12 L15.start
  constraint symmetric L3.end L12 L17.start
  constraint symmetric L4.end L12 L14.start
  constraint symmetric L5.end L12 L14.end
  constraint symmetric P0 L12 P1
  constraint symmetric L9.start L12 L13.start
  constraint symmetric L9.end L12 L13.end
  constraint symmetric L10.start L12 L16.start
  constraint symmetric L3.start L11 L29.start
  constraint symmetric L3.end L11 L29.end
  constraint symmetric L4.end L11 L33.end
  constraint symmetric L5.end L11 L31.end
  constraint symmetric P0 L11 P3
  constraint symmetric L9.start L11 L36.start
  constraint symmetric L9.end L11 L30.end
  constraint symmetric L10.start L11 L30.start
  constraint symmetric L11 P1 P2
  constraint symmetric L11 L14.end L23.end
  constraint symmetric L11 L15.start L25.start
  constraint symmetric L11 L14.start L23.start
  constraint symmetric L11 L13.start L22.start
  constraint symmetric L11 L13.end L21.end
  constraint symmetric L11 L17.start L24.start
  constraint symmetric L11 L16.start L21.start
  constraint horizontal L54
  constraint vertical L55
  constraint horizontal L56
  constraint vertical L57
  constraint horizontal L58
  constraint vertical L59
  constraint horizontal L60
  constraint vertical L61
  constraint horizontal L62
  constraint vertical L63
  constraint horizontal L64
  constraint vertical L65
  constraint horizontal L66
  constraint vertical L67
  constraint horizontal L68
  constraint vertical L69
  measures "d100" distance of L3 L9
extrude "Extrude12" add sketch "Sketch14" along normal blind 3 contours L3 L4 L5 L6 L9 L10 L54 L67 | L4 L19 L66 L67 L68 L69 | L5 L35 L54 L55 L56 L57 | L13 L14 L16 L18 L19 L20 L64 L69 | L29 L30 L32 L33 L35 L36 L56 L61 | L14 L23 L62 L63 L64 L65 | L26 L33 L58 L59 L60 L61 | L21 L22 L23 L25 L26 L27 L59 L62
chamfer "Chamfer3" distance 1 angle 45 4 edges at (62, 0, 8) (55, 7, 8) (48, 0, 8) (55, -7, 8)
sketch "Sketch17" plane through (0, 0, 0) normal (0, 0, -1) x (1, 0, 0)
  line L0 (30, -22.5) -> (25, -27.5)
  line L1 (25, -27.5) -> (25, -30)
  line L2 (25, -30) -> (-53, -30)
  line L3 (-53, -30) -> (-53, -27.5)
  line L4 (-53, -27.5) -> (-58, -22.5)
  line L5 (-58, -22.5) -> (-66, -22.5)
  line L6 (-66, -22.5) -> (-66, 22.5)
  line L7 (-66, 22.5) -> (-58, 22.5)
  line L8 (-58, 22.5) -> (-53, 27.5)
  line L9 (-53, 27.5) -> (-53, 30)
  line L10 (-53, 30) -> (25, 30)
  line L11 (25, 30) -> (25, 27.5)
  line L12 (25, 27.5) -> (30, 22.5)
  line L13 (30, 22.5) -> (66, 22.5)
  line L14 (66, 22.5) -> (66, -22.5)
  line L15 (66, -22.5) -> (30, -22.5)
  arc A0 (65, -35) -> (70, -30) centre (65, -30) ccw
  line L16 (70, -30) -> (70, 30)
  arc A1 (70, 30) -> (65, 35) centre (65, 30) ccw
  line L17 (65, 35) -> (-65, 35)
  arc A2 (-65, 35) -> (-70, 30) centre (-65, 30) ccw
  line L18 (-70, 30) -> (-70, -30)
  arc A3 (-70, -30) -> (-65, -35) centre (-65, -30) ccw
  line L19 (-65, -35) -> (65, -35)
  circle A4 centre (-56.6, 27.5) radius 2
  circle A5 centre (36.6, 27.5) radius 2
  circle A6 centre (36.6, -27.5) radius 2
  circle A7 centre (-66, 31) radius 2
  circle A8 centre (66, 31) radius 2
  circle A9 centre (-66, -31) radius 2
  circle A10 centre (66, -31) radius 2
  line L20 (40, 31) -> (-60, 31)
  line L21 (-60, 31) -> (-60, -31)
  line L22 (-60, -31) -> (40, -31)
  line L23 (40, -31) -> (40, 31)
  line L24 (40, 31) -> (-60, -31) construction
  line L25 (-60, 31) -> (40, -31) construction
  point P0 (-10, 0)
  dimension "d126" = 100
  dimension "d127" = 62
  constraint horizontal L20
  constraint perpendicular L20 L21
  constraint parallel L20 L22
  constraint parallel L21 L23
  constraint coincident L24 P0
  constraint coincident L25 P0
  measures "d126" distance of L21.end L22.end
  measures "d127" distance of L20.end L21.end
extrude "Extrude16" cut sketch "Sketch17" against normal blind 4 contours L0 L1 L2 L3 L4 L5 L15 L21 L22 L23 | L0 L1 L2 L3 L4 L5 L7 L8 L9 L10 L11 L12 L13 L15 L21 L23 | L7 L8 L9 L10 L11 L12 L13 L20 L21 L23
sketch "Sketch18" plane through (0, 0, 0) normal (0, 0, -1) x (1, 0, 0)
  circle A0 centre (66, -31) radius 2
  circle A1 centre (-66, -31) radius 2
  circle A2 centre (66, 31) radius 2
  circle A3 centre (-66, 31) radius 2
  arc A4 (65, -35) -> (70, -30) centre (65, -30) ccw
  line L0 (70, -30) -> (70, 30)
  arc A5 (70, 30) -> (65, 35) centre (65, 30) ccw
  line L1 (65, 35) -> (-65, 35)
  arc A6 (-65, 35) -> (-70, 30) centre (-65, 30) ccw
  line L2 (-70, 30) -> (-70, -30)
  arc A7 (-70, -30) -> (-65, -35) centre (-65, -30) ccw
  line L3 (-65, -35) -> (65, -35)
  line L4 (40, -22.5) -> (40, -31)
  line L5 (40, -31) -> (-60, -31)
  line L6 (-60, -31) -> (-60, -22.5)
  line L7 (-60, -22.5) -> (-66, -22.5)
  line L8 (-66, -22.5) -> (-66, 22.5)
  line L9 (-66, 22.5) -> (-60, 22.5)
  line L10 (-60, 22.5) -> (-60, 31)
  line L11 (-60, 31) -> (40, 31)
  line L12 (40, 31) -> (40, 22.5)
  line L13 (40, 22.5) -> (66, 22.5)
  line L14 (66, 22.5) -> (66, -22.5)
  line L15 (66, -22.5) -> (40, -22.5)
  line L16 (40, 22.5) -> (62, 22.5)
  line L17 (62, 22.5) -> (62, 31)
  line L18 (62, 31) -> (40, 31)
  line L19 (40, 31) -> (40, 22.5)
  line L20 (40, -22.5) -> (62, -22.5)
  line L21 (62, -22.5) -> (62, -31)
  line L22 (62, -31) -> (40, -31)
  line L23 (40, -31) -> (40, -22.5)
  dimension "d130" = 22
  dimension "d131" = 8.5
  dimension "d132" = 22
  dimension "d133" = 8.5
  constraint horizontal L16
  constraint vertical L17
  constraint horizontal L18
  constraint vertical L19
  constraint coincident L12.end L13.start
  constraint horizontal L20
  constraint vertical L21
  constraint horizontal L22
  constraint vertical L23
  constraint coincident L4.start L15.end
  measures "d130" distance of L12.end L16.end
  measures "d131" distance of L12.end L11.end
  measures "d132" distance of L4.start L20.end
  measures "d133" distance of L4.start L4.end
extrude "Extrude17" cut sketch "Sketch18" against normal blind 8 contours L4 L15 L20 L21 L22 L23 | L12 L13 L16 L17 L18 L19
chamfer "Chamfer5" distance 2 angle 45 6 edges at (1, -31, 0) (1, 31, 0) (62, -26.75, 0) (62, 26.75, 0) (64, 22.5, 0) (64, -22.5, 0)
extrude "Extrude18" cut 1 faces at (49.6667, 17.6667, 8) along direction (0, 0, 1) blind 3
sketch "Sketch20" plane through (0, 31, 0) normal (0, -1, 0) x (1, 0, 0)
  line L0 (-60, 2) -> (62, 2)
  line L1 (62, 2) -> (62, 11)
  line L2 (62, 11) -> (40, 11)
  line L3 (40, 11) -> (40, 4)
  line L4 (40, 4) -> (-60, 4)
  line L5 (-60, 4) -> (-60, 2)
  line L6 (41.6, 3.025) -> (60.4, 3.025)
  line L7 (60.4, 3.025) -> (60.4, 9.975)
  line L8 (60.4, 9.975) -> (41.6, 9.975)
  line L9 (41.6, 9.975) -> (41.6, 3.025)
  line L10 (41.6, 3.025) -> (60.4, 9.975) construction
  line L11 (60.4, 3.025) -> (41.6, 9.975) construction
  point P0 (51, 6.5)
  dimension "d142" = 18.8
  dimension "d143" = 6.95
  dimension "d144" = 11
  dimension "d145" = 4.5
  constraint horizontal L6
  constraint perpendicular L6 L7
  constraint parallel L6 L8
  constraint parallel L7 L9
  constraint coincident L10 P0
  constraint coincident L11 P0
  measures "d142" distance of L7.end L8.end
  measures "d143" distance of L6.end L7.end
  measures "d144" distance of L3 P0
  measures "d145" distance of L2 P0
extrude "Extrude19" cut sketch "Sketch20" against normal blind 7 contours L6 L7 L8 L9
